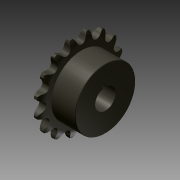
# Autodesk Inventor part: i-Sprocket
Saved by Autodesk Inventor 2015 (Build 190159000, 159)
## iProperties
Category: iParts
Company: FirstCadLibrary
Shininess: 64.0
Length Units: 11272
Angle Units: 11279
Time Units: 11290
Mass Units: 11286
Length Display Precision: 3
Angle Display Precision: 2
Compacted: True
Part Number: i-Sprocket
Document SubType Name: Modeling
Created: 2006-02-06
Designer: Ed Sparks
Material: Steel, Mild
Engineer: Ed Sparks
Density: 7.86 g/cm^3
Appearance: Gunmetal
Density: 0.0
Volumn: 0.0
Area: 0.0
PropertySet Name: Model Information
Control State: 0
Master: False
Checked Out: False
Title: i-Sprocket
Subject: i-Sprocket
Author: Ed Sparks
Keywords: Sprocket
Autodesk Inventor part; units mm, degrees
ref_plane "YZ Plane" through (0, 0, 0) normal (1, 0, 0) x (0, 1, 0)
ref_plane "XZ Plane" through (0, 0, 0) normal (0, 1, 0) x (-1, 0, 0)
ref_plane "XY Plane" through (0, 0, 0) normal (0, 0, 1) x (1, 0, 0)
sketch "Sketch1" plane through (0, 0, 0) normal (0, 0, 1) x (1, 0, 0)
  line L0 (-2.1384, 0) -> (2.1384, 0)
  line L1 (0, 0) -> (0, 26.8002) construction
  line L2 (-0.9484, 26.8002) -> (0.9484, 26.8002)
  line L3 (-2.1384, 0) -> (-2.1384, 22.0377)
  line L4 (2.1384, 0) -> (2.1384, 22.0377)
  arc A0 (-0.9484, 26.8002) -> (-2.1384, 22.0377) centre (7.9867, 22.0377) ccw
  arc A1 (2.1384, 22.0377) -> (0.9484, 26.8002) centre (-7.9867, 22.0377) ccw
  point P0 (25.317, 18.8926)
  dimension "d0" = 4.2767
  dimension "d1" = 26.8002
  dimension "d2" = 4.7625
  dimension "d3" = 10.1251
  constraints: 10 end point, 4 point on circle, 2 centre point, 2 coincident, 2 horizontal, 2 horizontal alignment, 2 midpoint, 2 parallel, 2 perpendicular, 2 symmetric about line, 1 other
  measures "d0" distance of L0.start L0.end
  measures "d1" distance between parallel lines of L0 L2
  measures "d2" distance from line of point (7.987, 22.038) L2
  measures "d3" distance of point (7.987, 22.038) L3.end
revolve "Sprocket Blank" add sketch "Sketch1" angle 360 about axis through (-2.1384, 0, 0) along (1, 0, 0)
sketch "Sketch2" plane through (2.1384, 0, 0) normal (1, 0, 0) x (0, 0, -1)
  circle A0 centre (0, 0) radius 22.0377 projected
  line L0 (0, 0) -> (0, 35.1967) construction
  circle A1 centre (0, 0) radius 24.4118 construction
  line L1 (0, 0) -> (7.0581, 35.4835) construction
  arc A2 (-2.0205, 22.7901) -> (2.0205, 22.7901) centre (0, 24.4118) ccw
  arc A3 (2.0205, 22.7901) -> (3.0338, 24.5459) centre (-3.1695, 26.9555) ccw
  arc A4 (-3.0338, 24.5459) -> (-2.0205, 22.7901) centre (3.1695, 26.9555) ccw
  line L2 (0, 0) -> (-6.8144, 34.2581) construction
  arc A5 (-3.0338, 24.5459) -> (-5.3509, 26.9009) centre (-6.9255, 23.0342) ccw
  arc A6 (5.3509, 26.9009) -> (3.0338, 24.5459) centre (6.9255, 23.0342) ccw
  arc A7 (5.3509, 26.9009) -> (-5.3509, 26.9009) centre (0, 0) ccw
  dimension "d9" = 48.8235
  dimension "d10" = 11.25
  dimension "d11" = 6.9255
  dimension "d12" = 3.1694
  dimension "d13" = 1.3776
  dimension "d15" = 2.5438
  dimension "d17" = 5.1816
  constraints: 14 coincident, 12 point on circle, 6 centre point, 6 end point, 3 point on line, 3 tangent, 2 horizontal alignment, 2 symmetric about line, 1 vertical, 1 vertical alignment, 5 other
  measures "d10" angle of L1 L0
  measures "d11" horizontal distance of point (6.926, 23.034) L0.start
  measures "d12" horizontal distance of point (-3.169, 26.956) L0.start
  measures "d13" vertical distance of point (6.926, 23.034) point (0, 24.412)
  measures "d15" vertical distance of point (0, 24.412) point (-3.169, 26.956)
  measures "d17" diameter of A2
extrude "Tooth Profile" cut sketch "Sketch2" against normal blind 25.4 contours A2 A0 | A0 A2 A4 A5 A7 A6 A3 picked at (0, 21.9638)
sketch "Sketch4" plane through (2.1384, 0, 0) normal (1, 0, 0) x (0, 0, -1)
  arc A0 (0, -2.5897) -> (0, -2.5897) centre (0, 0) ccw
  circle A1 centre (0, 0) radius 18.6531
  arc A2 (-0.9854, 22.0157) -> (0.9854, 22.0157) centre (0, 0) ccw projected
  dimension "d23" = 37.3062
  constraints: 2 centre point, 2 coincident, 2 point on circle, 1 concentric
  measures "d23" diameter of A1
extrude "Hub" add sketch "Sketch4" along normal blind 14.7733 contours A0 | A1
sketch "Sketch5" plane through (-2.1384, 0, 0) normal (-1, 0, 0) x (0, 0, 1)
  circle A0 centre (0, 0) radius 22.0377 projected
  constraints: 1 coincident
hole "Bore" at (-2.1384, 0, 0) direction (1, 0, 0) diameter 12.7 end through all
sketch "Sketch6" plane through (-2.1384, 0, 0) normal (-1, 0, 0) x (0, 0, 1)
  circle A0 centre (0, 0) radius 6.35 projected
  circle A1 centre (0, 0) radius 22.0377 projected
  line L0 (-1.5875, 4.7625) -> (1.5875, 4.7625)
  line L1 (1.5875, 4.7625) -> (1.5875, 7.9375)
  line L2 (1.5875, 7.9375) -> (-1.5875, 7.9375)
  line L3 (-1.5875, 7.9375) -> (-1.5875, 4.7625)
  line L4 (0, 0) -> (0, 24.369) construction
  dimension "d49" = 3.175
  dimension "d50" = 7.9375
  constraints: 10 end point, 3 parallel, 2 equal length, 1 horizontal, 1 perpendicular, 1 other
  measures "d49" distance of L1.end L2.end
  measures "d50" distance from line of A0.centre L2
extrude "Keyway" cut sketch "Sketch6" against normal through all contours L1 L0 L3 A0 | A0 L3 L2 L1 picked at (0.1781, 5.2842)
sketch "Sketch7" plane through (2.1384, 0, 0) normal (1, 0, 0) x (0, 0, -1)
  circle A0 centre (0, 0) radius 13.4938
  arc A1 (0, 14.3146) -> (0, 14.3146) centre (0, 0) ccw
  circle A2 centre (0, 0) radius 16.1131
  circle A3 centre (0, 0) radius 18.6531 projected
  circle A4 centre (0, 0) radius 18.6531 projected
  dimension "d39" = 32.2263
  constraints: 3 centre point, 3 coincident, 2 point on circle, 1 concentric
  measures "d39" diameter of A2
extrude "Undercut" [suppressed]
chamfer "Hub_Chamfer" distance 0.254 angle 45 1 edges at (16.9116, 0, 18.6531)
pattern_circular "Circular Pattern2" count 16 over 360 about axis through (-10, 0, 0) along (1, 0, 0) of "Tooth Profile"
equation "\"d0\" = Sprocket_Thickness"
equation "\"d1\" = Outside_Radius"
equation "\"d2\" = Depth_Of_Chamfer"
equation "\"d3\" = Chamfer_Radius"
equation "\"d9\" = Pitch_Diameter"
equation "\"d11\" = W_"
equation "\"d12\" = M_"
equation "\"d13\" = V_"
equation "\"d15\" = T_"
equation "\"d17\" = Seating_Curve_Diameter"
equation "\"d23\" = Hub_Diameter"
equation "\"d24\" = Length_Through_Bore - Sprocket_Thickness"
equation "\"d42\" = Bore_Diameter"
equation "\"d49\" = Key_Width"
equation "\"d50\" = 0.5 * Bore_Diameter + 0.5 * Key_Width"
equation "\"d37\" = Hub_Chamfer"
equation "\"Chamfer_Radius\" = 1.063 * Chain_Pitch"
equation "\"Depth_Of_Chamfer\" = 0.5 * Chain_Pitch"
equation "\"Chain_Pitch\" = 9.525"
equation "\"Roller_Diameter\" = 5.08"
equation "\"d14\" = F_"
equation "\"d16\" = E_"
equation "\"Hub_Diameter\" = 37.30625"
equation "\"Bore_Diameter\" = 12.7"
equation "\"Length_Through_Bore\" = 19.05"
equation "\"Key_Width\" = 3.175"
equation "\"Hub_Chamfer\" = 0.254"
equation "\"Sprocket_Thickness\" = 4.276725"
equation "\"Outside_Radius\" = 26.800204"
equation "\"Pitch_Diameter\" = 48.823539"
equation "\"Seating_Curve_Diameter\" = 5.1816"
equation "\"F_\" = 4.209472"
equation "\"E_\" = 6.6548"
equation "\"W_\" = 6.925521"
equation "\"M_\" = 3.169451"
equation "\"V_\" = 1.377572"
equation "\"T_\" = 2.543753"
body "Solid1"
